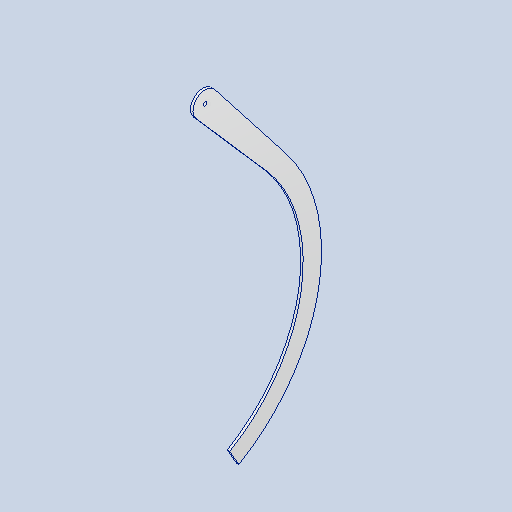
# Autodesk Inventor part: hand-grab-v5-Plate-4
Saved by Autodesk Inventor 2025.2 (Build 292293000, 293)
## iProperties
Created: 2025-05-11
Part Number: hand-grab-v5-Plate-4
Material: アルミニウム 6061
Document SubType Name: Modeling
Designer: haruy
Density: 2.7 g/cm^3
Appearance: アルミニウム - フラット
Author: haruy
Autodesk Inventor part; units mm, degrees
ref_plane "YZ Plane" through (0, 0, 0) normal (1, 0, 0) x (0, 1, 0)
ref_plane "XZ Plane" through (0, 0, 0) normal (0, 1, 0) x (-1, 0, 0)
ref_plane "XY Plane" through (0, 0, 0) normal (0, 0, 1) x (1, 0, 0)
derived "hand-grab-v5-Sketch-Base.ipt"
sketch "スケッチ1" plane through (0, 0, 0) normal (1, 0, 0) x (0, 1, 0)
  circle A0 centre (0, 0) radius 120 construction
  line L0 (196.3075, 10) -> (258.3075, 10)
  line L1 (258.3075, 10) -> (258.3075, -10)
  line L2 (258.3075, -10) -> (196.3075, -10)
  line L3 (196.3075, -10) -> (196.3075, 10)
  line L4 (196.3075, 5) -> (188.3075, 5)
  line L5 (188.3075, 5) -> (188.3075, -5)
  line L6 (188.3075, -5) -> (196.3075, -5)
  line L7 (196.3075, -5) -> (196.3075, 5)
  line L8 (188.3075, 2.5) -> (168.3075, 2.5)
  line L9 (168.3075, 2.5) -> (168.3075, -2.5)
  line L10 (168.3075, -2.5) -> (188.3075, -2.5)
  line L11 (188.3075, -2.5) -> (188.3075, 2.5)
  line L12 (183.3075, 2.5) -> (183.3075, -2.5)
  line L13 (183.3075, 4.619) -> (179.3075, 4.619)
  line L14 (179.3075, 4.619) -> (179.3075, -4.619)
  line L15 (179.3075, -4.619) -> (183.3075, -4.619)
  line L16 (183.3075, -4.619) -> (183.3075, 4.619)
  circle A1 centre (0, 0) radius 135 construction
  line L17 (290.4898, -280) -> (-352.5984, -280)
  circle A2 centre (151.819, -40) radius 25
  line L18 (0, 0) -> (-116.9134, -67.5) construction
  line L19 (0, 0) -> (-135, 0)
  line L20 (-118.3216, -20) -> (-133.5103, -20)
  circle A3 centre (151.819, -40) radius 10
  line L21 (78.9419, -90.3779) -> (145.2405, -32.4685)
  line L22 (157.9765, -47.8794) -> (83.126, -106.3723)
  line L23 (0, 0) -> (0, -280)
  circle A4 centre (151.819, -40) radius 256.5229
  line L24 (151.819, -40) -> (-103.923, -60)
  line L25 (151.819, -40) -> (0, -120)
  line L26 (151.819, -40) -> (-49.0169, -199.5899)
  line L27 (179.3075, 17) -> (142.3945, 17)
  line L28 (142.3945, 17) -> (142.3945, -12.5)
  line L29 (142.3945, -12.5) -> (179.3075, -12.5)
  line L30 (179.3075, -12.5) -> (179.3075, 17)
  line L31 (174.3075, 2.5) -> (174.3075, -2.5)
  line L32 (174.3075, 5) -> (170.3075, 5)
  line L33 (170.3075, 5) -> (170.3075, -5)
  line L34 (170.3075, -5) -> (174.3075, -5)
  line L35 (174.3075, -5) -> (174.3075, 5)
  line L36 (166.3075, 8) -> (174.3075, 8)
  line L37 (174.3075, 8) -> (174.3075, -8)
  line L38 (174.3075, -8) -> (166.3075, -8)
  line L39 (166.3075, -8) -> (166.3075, 8)
  line L40 (179.3075, -12.5) -> (142.3945, -12.5)
  line L41 (142.3945, -12.5) -> (142.3945, -17)
  line L42 (142.3945, -17) -> (179.3075, -17)
  line L43 (179.3075, -17) -> (179.3075, -12.5)
  line L44 (144.7515, -17) -> (143.1795, -12.5)
  line L45 (143.1795, -12.5) -> (141.6095, -12.5)
  line L46 (141.6095, -12.5) -> (140.0375, -17)
  line L47 (140.0375, -17) -> (144.7515, -17)
  line L48 (149.4625, -12.5) -> (147.8925, -12.5)
  line L49 (151.0345, -17) -> (149.4625, -12.5)
  line L50 (147.8925, -12.5) -> (146.3205, -17)
  line L51 (146.3205, -17) -> (151.0345, -17)
  line L52 (155.7455, -12.5) -> (154.1755, -12.5)
  line L53 (157.3175, -17) -> (155.7455, -12.5)
  line L54 (154.1755, -12.5) -> (152.6035, -17)
  line L55 (152.6035, -17) -> (157.3175, -17)
  line L56 (162.0285, -12.5) -> (160.4585, -12.5)
  line L57 (163.6005, -17) -> (162.0285, -12.5)
  line L58 (160.4585, -12.5) -> (158.8865, -17)
  line L59 (158.8865, -17) -> (163.6005, -17)
  line L60 (168.3115, -12.5) -> (166.7415, -12.5)
  line L61 (169.8835, -17) -> (168.3115, -12.5)
  line L62 (166.7415, -12.5) -> (165.1695, -17)
  line L63 (165.1695, -17) -> (169.8835, -17)
  line L64 (174.5945, -12.5) -> (173.0245, -12.5)
  line L65 (176.1665, -17) -> (174.5945, -12.5)
  line L66 (173.0245, -12.5) -> (171.4525, -17)
  line L67 (171.4525, -17) -> (176.1665, -17)
  line L68 (151.0345, -17) -> (152.6035, -17)
  line L69 (143.1795, -12.5) -> (143.1795, 28.2865)
  line L70 (171.4525, -17) -> (169.8835, -17)
  line L71 (180.8775, -12.5) -> (179.3075, -12.5)
  line L72 (182.4495, -17) -> (180.8775, -12.5)
  line L73 (179.3075, -12.5) -> (177.7355, -17)
  line L74 (177.7355, -17) -> (182.4495, -17)
  line L75 (179.3075, -15) -> (142.3945, -15)
  circle A5 centre (151.819, -40) radius 27
  line L76 (120, 148.4359) -> (120, -215.0589)
  arc A6 (-103.923, -60) -> (78.9419, -90.3779) centre (0, 0) ccw
  arc A7 (-116.9134, -67.5) -> (83.126, -106.3723) centre (0, 0) ccw
  line L77 (-103.923, -60) -> (-116.9134, -67.5)
  line L78 (119.5722, -122.5175) -> (142.1536, -37.4348)
  line L79 (161.3299, -43.0891) -> (131.9849, -133.4377)
  arc A8 (-49.0169, -199.5899) -> (119.5722, -122.5175) centre (3.5876, -91.7346) ccw
  line L80 (-49.0169, -199.5899) -> (-55.5925, -213.0718)
  circle A9 centre (3.5876, -91.7346) radius 135 construction
  arc A10 (-55.5925, -213.0718) -> (131.9849, -133.4377) centre (3.5876, -91.7346) ccw
  line L81 (191.3075, 72) -> (196.3075, 72)
  line L82 (196.3075, 72) -> (196.3075, -72)
  line L83 (196.3075, -72) -> (191.3075, -72)
  line L84 (191.3075, -72) -> (191.3075, 72)
  line L85 (196.3075, -72) -> (156.819, -72)
  line L86 (156.819, -72) -> (156.819, -77)
  line L87 (156.819, -77) -> (196.3075, -77)
  line L88 (196.3075, -77) -> (196.3075, -72)
  line L89 (143.1795, 0) -> (179.3075, 0)
  circle A11 centre (151.819, -40) radius 8.25 construction
  circle A12 centre (151.819, -40) radius 13.25
  line L90 (156.819, -72) -> (140.7102, -47.2221)
  line L91 (144.8498, -28.7309) -> (191.3075, 0)
  circle A13 centre (193.8075, 0) radius 1.5
  circle A14 centre (193.8075, -36) radius 1.5
  line L92 (144.8498, 28.7309) -> (191.3075, 0)
  circle A15 centre (193.8075, 36) radius 1.5
  line L93 (196.3075, 72) -> (156.819, 72)
  line L94 (156.819, 72) -> (140.7102, 47.2221)
  circle A16 centre (151.819, 40) radius 13.25
  circle A17 centre (151.819, 40) radius 7.5
  circle A18 centre (151.819, -40) radius 7.5
  circle A19 centre (151.819, -40) radius 1.5
  line L95 (151.819, -40) -> (151.819, -179.6263)
  point P0 (188.3075, 0)
  point P1 (142.3945, -12.5)
  point P2 (151.819, -17)
  point P3 (151.819, -17)
  point P4 (170.668, -17)
  point P5 (183.5696, -15)
  point P6 (174.3075, 0)
  point P7 (141.4453, -48.2432)
  point P8 (141.3984, -48.2805)
  point P9 (151.819, -52.6913)
  dimension "d1" = 3
  measures "d1" diameter of A19
extrude "押し出し1" add sketch "スケッチ1" against normal blind 2 contours A5 L78 A2 L22 | L22 L78 A5 | A3 L95 A18 L24 | A2 L78 L26 L90 L22 | L22 L76 L26 A5 L78 | A5 L26 A2 L78 | L90 L26 A12 L22 | L22 L95 A3 | A12 L26 A3 L95 L22 | L22 A7 L26 L76 | A2 L26 L78 | A5 L25 A2 L26 | L26 L76 L25 A5 | L90 A12 L26 | L26 L78 L25 A12 L90 | A12 L24 L21 | L21 A3 L78 L24 A12 | A3 L26 A18 L95 | A12 L25 A3 L26 | L26 A7 L23 A6 L21 L25 L76 | A2 L25 L78 L26 | A5 L21 A2 L25 | L25 L76 L21 A5 | L24 A12 L78 L25 A2 L21 | L24 L78 A12 | A3 L25 A18 L26 | L95 A19 L24 A18 | A18 L26 A19 L95 | A3 L24 L78 | L25 L21 L76 | A7 A4 A6 L23 | A7 L77 A4 | L78 A12 L25 | A12 L78 L24 A3 L25 | A3 L24 A18 L25 | A18 L25 A19 L26 | A18 L24 A19 L25
